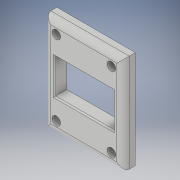
# Autodesk Inventor part: Molex Mount
Saved by Autodesk Inventor 2017 (Build 210142000, 142)
## iProperties
Created: 2017-02-12
Part Number: Molex Mount
Material: Generic
Document SubType Name: Modeling
Designer: Roksbot
Density: 1 g/cm^3
Appearance: Default
Author: Roksbot
Autodesk Inventor part; units mm, degrees
ref_plane "YZ Plane" through (0, 0, 0) normal (1, 0, 0) x (0, 1, 0)
ref_plane "XZ Plane" through (0, 0, 0) normal (0, 1, 0) x (-1, 0, 0)
ref_plane "XY Plane" through (0, 0, 0) normal (0, 0, 1) x (1, 0, 0)
sketch "Sketch1" plane through (0, 0, 0) normal (0, 0, 1) x (1, 0, 0)
  line L0 (20.32, -25.4) -> (-20.32, -25.4)
  line L1 (-20.32, -25.4) -> (-20.32, 25.4)
  line L2 (-20.32, 25.4) -> (20.32, 25.4)
  line L3 (20.32, 25.4) -> (20.32, -25.4)
  line L4 (20.32, -25.4) -> (-20.32, 25.4) construction
  line L5 (-20.32, -25.4) -> (20.32, 25.4) construction
  line L6 (15.24, -9.017) -> (-15.24, -9.017)
  line L7 (-15.24, -9.017) -> (-15.24, 9.017)
  line L8 (-15.24, 9.017) -> (15.24, 9.017)
  line L9 (15.24, 9.017) -> (15.24, -9.017)
  line L10 (15.24, -9.017) -> (-15.24, 9.017) construction
  line L11 (-15.24, -9.017) -> (15.24, 9.017) construction
  point P0 (0, 0)
  point P1 (0, 0)
  point P2 (0, 0)
  point P3 (0, 0)
  point P4 (0, 0)
  dimension "d0" = 40.64
  dimension "d1" = 30.48
  dimension "d3" = 50.8
  dimension "d4" = 18.034
  constraints: 24 end point, 8 midpoint, 4 parallel, 2 horizontal, 2 perpendicular, 1 coincident
  measures "d0" distance of L1.end L2.end
  measures "d1" distance of L7.end L8.end
  measures "d3" distance of L0.end L1.end
  measures "d4" distance of L8.end L6.start
extrude "Extrusion1" add sketch "Sketch1" along normal blind 6.35
sketch "Sketch2" plane through (0, 0, 6.35) normal (0, 0, 1) x (1, 0, 0)
  circle A0 centre (-14.2875, -19.3675) radius 2.2225
  circle A1 centre (14.2875, -19.3675) radius 2.2225
  line L0 (-20.32, -25.4) -> (20.32, -25.4) projected
  line L1 (-15.24, -9.017) -> (-15.24, 9.017) projected
  line L2 (-15.24, 9.017) -> (15.24, 9.017) projected
  line L3 (15.24, 9.017) -> (15.24, -9.017) projected
  line L4 (15.24, -9.017) -> (-15.24, -9.017) projected
  line L5 (-20.32, -25.4) -> (20.32, -25.4) projected
  line L6 (20.32, -25.4) -> (20.32, 25.4) projected
  line L7 (20.32, 25.4) -> (-20.32, 25.4) projected
  line L8 (-20.32, 25.4) -> (-20.32, -25.4) projected
  circle A2 centre (-14.2875, 19.3675) radius 2.2225
  circle A3 centre (14.2875, 19.3675) radius 2.2225
  point P0 (0, 0)
  dimension "d7" = 4.445
  dimension "d8" = 3.81
  dimension "d10" = 3.81
  dimension "d11" = 3.81
  dimension "d18" = 3.81
  constraints: 4 centre point, 3 equal radius, 2 horizontal alignment, 2 vertical alignment
  measures "d7" diameter of A0
  measures "d8" distance edge to line of A0 L0
  measures "d10" distance edge to line of A1 L6
  measures "d11" distance edge to line of A0 L8
  measures "d18" distance edge to line of A2 L7
extrude "Extrusion2" cut sketch "Sketch2" against normal through all contours A0 | A1 | A2 | A3
fillet "Fillet1" radius 3.175 4 edges at (-20.32, 0, 6.35) (0, 25.4, 6.35) (20.32, 0, 6.35) (0, -25.4, 6.35)
chamfer "Chamfer1" distance 0.635 angle 45 4 edges at (-15.24, 0, 6.35) (0, 9.017, 6.35) (15.24, 0, 6.35) (0, -9.017, 6.35)
equation "\"d10\" = d11"
equation "\"d11\" = d8"
equation "\"d18\" = d8"
body "Solid1"
